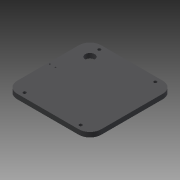
# Autodesk Inventor part: board
Saved by Autodesk Inventor 2013 (Build 170138000, 138)
## iProperties
Created: 2013-07-23
Part Number: board
Material: Generic
Document SubType Name: Modeling
Designer: employee
Density: 1 g/cm^3
Mass: 551.733 g
Surface Area: 1133 cm^2
Volume: 551.733 cm^3
Author: employee
Autodesk Inventor part; units mm, degrees
ref_plane "YZ Plane" through (0, 0, 0) normal (1, 0, 0) x (0, 1, 0)
ref_plane "XZ Plane" through (0, 0, 0) normal (0, 1, 0) x (-1, 0, 0)
ref_plane "XY Plane" through (0, 0, 0) normal (0, 0, 1) x (1, 0, 0)
sketch "Sketch1" plane through (0, 0, 0) normal (0, 0, 1) x (1, 0, 0)
  circle A0 centre (0, 0) radius 100 construction
  line L0 (112.5, 0) -> (112.5, 112.5)
  line L1 (112.5, 112.5) -> (-112.5, 112.5)
  line L2 (-112.5, 112.5) -> (-112.5, -112.5)
  line L3 (-112.5, -112.5) -> (112.5, -112.5)
  line L4 (112.5, -112.5) -> (112.5, 0)
  circle A1 centre (-75, -100) radius 4.05
  circle A2 centre (75, -100) radius 4.05
  line L5 (75, -100) -> (-75, -100) construction
  line L6 (-75, -100) -> (-75, 100) construction
  line L7 (-75, 100) -> (75, 100) construction
  line L8 (75, 100) -> (75, -100) construction
  circle A3 centre (-75, 100) radius 4.05
  circle A4 centre (75, 100) radius 4.05
  point P0 (0, 112.5)
  point P1 (75, 0)
  dimension "d0" = 200
  dimension "d2" = 225
  dimension "d3" = 225
  dimension "d4" = 150
  dimension "d5" = 37.5
  dimension "d6" = 12.5
  dimension "d7" = 8.1
  constraints: 18 end point, 5 centre point, 4 coincident, 4 parallel, 3 equal radius, 3 horizontal alignment, 2 collinear, 2 midpoint, 2 perpendicular, 1 horizontal, 1 vertical, 1 vertical alignment
  measures "d0" diameter of A0
  measures "d2" distance of L0.end L1.end
  measures "d3" distance between parallel lines of L3 L1
  measures "d4" distance of L5.start A1.centre
  measures "d5" distance from line of A1.centre L2
  measures "d6" distance from line of A1.centre L3
  measures "d7" diameter of A1
extrude "Extrusion1" add sketch "Sketch1" along normal blind 12.7
fillet "Fillet1" radius 30 4 edges at (-112.5, -112.5, 6.35) (-112.5, 112.5, 6.35) (112.5, -112.5, 6.35) (112.5, 112.5, 6.35)
sketch "Sketch2" plane through (0, 0, 0) normal (0, 0, -1) x (-1, 0, 0)
  circle A0 centre (0, 0) radius 100
  dimension "d14" = 200
  constraints: 1 centre point, 1 coincident
  measures "d14" diameter of A0
extrude "Extrusion2" cut sketch "Sketch2" against normal blind 2
sketch "Sketch4" plane through (0, 0, 0) normal (0, 0, -1) x (-1, 0, 0)
  circle A0 centre (92.5, 0) radius 1.55
  circle A1 centre (107.5, 0) radius 1.55
  circle A2 centre (0, 0) radius 100 projected
  line L0 (112.5, 82.5) -> (112.5, -82.5) projected
  dimension "d44" = 15
  dimension "d45" = 0
  dimension "d46" = 5
  dimension "d47" = 3.1
  constraints: 2 centre point, 1 equal radius, 1 horizontal alignment
  measures "d44" distance of A1.centre A0.centre
  measures "d45" vertical distance of A0.centre A2.centre
  measures "d46" distance from line of L0 A1.centre
  measures "d47" diameter of A1
hole "Hole1" at (-92.5, 0, 0) at (-107.5, 0, 0) direction (0, 0, 1) diameter 3.4 end through all counterbore diameter 6.5 counterbore depth 4.5 clearance for "Socket Head Cap Screw" size "M3" standard "Ansi Metric M Profile"
sketch "Sketch5" plane through (0, 0, 2) normal (0, 0, -1) x (-1, 0, 0)
  circle A0 centre (0, 0) radius 100 projected
  circle A1 centre (70.7107, 70.7107) radius 12.5
  line L0 (0, 0) -> (70.7107, 70.7107) construction
  line L1 (82.5, -112.5) -> (-82.5, -112.5) construction
  dimension "d32" = 25
  dimension "d35" = 45
  constraints: 2 end point, 1 centre point, 2 other
  measures "d32" diameter of A1
  measures "d35" angle of L1 L0
extrude "Extrusion4" cut sketch "Sketch5" along normal through all both and the other way through all contours A1 A0 | A0 A1 picked at (68.0843, 67.4022) picked at (73.7867, 73.4347)
sketch "Sketch6" plane through (0, 0, 2) normal (0, 0, -1) x (-1, 0, 0)
  arc A0 (61.3367, 78.9798) -> (78.9798, 61.3367) centre (70.7107, 70.7107) ccw projected
  arc A1 (61.3367, 78.9798) -> (78.9798, 61.3367) centre (0, 0) ccw projected
  arc A2 (27.6392, 96.1045) -> (96.1045, 27.6392) centre (70.7107, 70.7107) ccw
  dimension "d39" = 50
  constraints: 4 point on circle, 1 centre point, 1 coincident
  measures "d39" radius of A2
extrude "Extrusion5" cut sketch "Sketch6" against normal blind 3 contours A0 A1 A2
body "Solid1"
